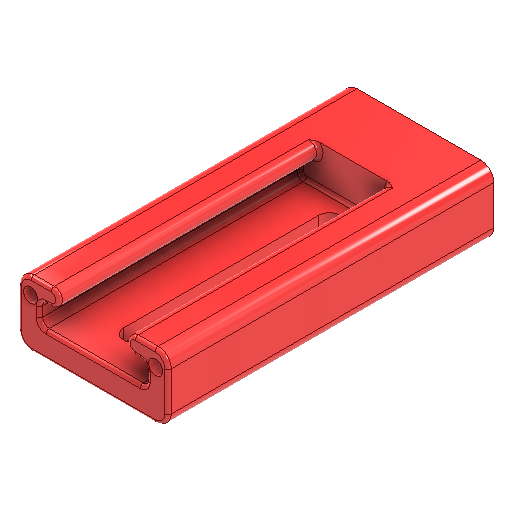
# Autodesk Inventor part: VerticalProfile
Saved by Autodesk Inventor 2023 (Build 270158000, 158)
## iProperties
Created: 2024-05-30
Part Number: VerticalProfile
Material: Generic
Document SubType Name: Modeling
Designer: Sven
Density: 1 g/cm^3
Appearance: Light Red
Author: Sven
Autodesk Inventor part; units mm, degrees
ref_plane "YZ Plane" through (0, 0, 0) normal (1, 0, 0) x (0, 1, 0)
ref_plane "XZ Plane" through (0, 0, 0) normal (0, 1, 0) x (-1, 0, 0)
ref_plane "XY Plane" through (0, 0, 0) normal (0, 0, 1) x (1, 0, 0)
sketch "Sketch1" plane through (0, 0, 0) normal (0, 0, 1) x (1, 0, 0)
  circle A0 centre (-4.5, -25.25) radius 1.65 projected
  circle A1 centre (4.5, -25.25) radius 1.65 projected
  arc A2 (25.5, 29.25) -> (23.5, 31.25) centre (23.5, 29.25) ccw projected
  line L0 (23.5, 31.25) -> (-23.5, 31.25) projected
  arc A3 (-23.5, 31.25) -> (-25.5, 29.25) centre (-23.5, 29.25) ccw projected
  line L1 (-25.5, 29.25) -> (-25.5, -29.25) projected
  arc A4 (-25.5, -29.25) -> (-23.5, -31.25) centre (-23.5, -29.25) ccw projected
  line L2 (-23.5, -31.25) -> (23.5, -31.25) projected
  arc A5 (23.5, -31.25) -> (25.5, -29.25) centre (23.5, -29.25) ccw projected
  line L3 (25.5, -29.25) -> (25.5, 29.25) projected
  line L4 (9.5, -21.25) -> (-9.5, -21.25)
  line L5 (-11.5, -23.25) -> (-11.5, -29.25)
  line L6 (-9.5, -31.25) -> (9.5, -31.25)
  line L7 (11.5, -29.25) -> (11.5, -23.25)
  circle A6 centre (4.5, -25.25) radius 2
  circle A7 centre (-4.5, -25.25) radius 2
  arc A8 (11.5, -23.25) -> (9.5, -21.25) centre (9.5, -23.25) ccw
  arc A9 (-9.5, -21.25) -> (-11.5, -23.25) centre (-9.5, -23.25) ccw
  arc A10 (-11.5, -29.25) -> (-9.5, -31.25) centre (-9.5, -29.25) ccw
  arc A11 (9.5, -31.25) -> (11.5, -29.25) centre (9.5, -29.25) ccw
  circle A12 centre (9.6, -23.75) radius 1.1 projected
  circle A13 centre (-9.6, -23.75) radius 1.1 projected
  point P0 (0, 0)
  point P1 (-11.5, -31.25)
  point P2 (0, -21.25)
  point P3 (0, -31.25)
  dimension "d0" = 23
  dimension "d1" = 10
  dimension "d2" = 4
  dimension "d3" = 4
  dimension "d4" = 2
  dimension "d5" = 2
  constraints: 8 end point, 8 point on circle, 8 tangent, 6 centre point, 3 point on line, 2 coincident, 2 equal radius, 2 midpoint, 2 parallel, 1 horizontal, 1 perpendicular, 1 vertical alignment
  measures "d0" distance between parallel lines of L5 L7
  measures "d1" distance between parallel lines of L6 L4
  measures "d2" diameter of A6
  measures "d3" diameter of A7
  measures "d4" radius of A8
  measures "d5" radius of A9
extrude "Extrusion1" add sketch "Sketch1" along normal blind 6 contours L2 A10 L5 A9 L4 A8 L7 A11 | A12 | A13
sketch "Sketch2" plane through (0, 0, 6) normal (0, 0, 1) x (1, 0, 0)
  arc A0 (-11.5, -29.25) -> (-9.5, -31.25) centre (-9.5, -29.25) ccw projected
  line L0 (-9.5, -31.25) -> (9.5, -31.25) projected
  arc A1 (9.5, -31.25) -> (11.5, -29.25) centre (9.5, -29.25) ccw projected
  line L1 (11.5, -29.25) -> (11.5, -23.25) projected
  arc A2 (11.5, -23.25) -> (9.5, -21.25) centre (9.5, -23.25) ccw projected
  line L2 (9.5, -21.25) -> (-9.5, -21.25) projected
  arc A3 (-9.5, -21.25) -> (-11.5, -23.25) centre (-9.5, -23.25) ccw projected
  line L3 (-11.5, -23.25) -> (-11.5, -29.25) projected
  circle A4 centre (-4.5, -25.25) radius 2 projected
  circle A5 centre (4.5, -25.25) radius 2 projected
  point P0 (0, 0)
extrude "Extrusion2" add sketch "Sketch2" along normal blind 4 contours L3 A3 L2 A2 L1 A1 L0 A0 | A4 | A5
sketch "Sketch3" plane through (0, 0, 10) normal (0, 0, 1) x (1, 0, 0)
  line L0 (9.5, -21.25) -> (-9.5, -21.25) projected
  arc A0 (6.45, -21.25) -> (6.45, -23.75) centre (6.45, -22.5) ccw
  arc A1 (-6.45, -23.75) -> (-6.45, -21.25) centre (-6.45, -22.5) ccw
  line L1 (9.5, -21.25) -> (-9.5, -21.25) projected
  line L2 (6.45, -23.75) -> (-6.45, -23.75)
  line L3 (-9.5, -31.25) -> (9.5, -31.25) projected
  line L4 (7.25, -27.25) -> (-7.25, -27.25)
  line L5 (8.25, -26.25) -> (8.25, -24.75)
  line L6 (11.5, -29.25) -> (11.5, -23.25) projected
  line L7 (-8.25, -26.25) -> (-8.25, -24.75)
  line L8 (-11.5, -23.25) -> (-11.5, -29.25) projected
  line L9 (6.45, -23.75) -> (7.25, -23.75)
  line L10 (-6.45, -23.75) -> (-7.25, -23.75)
  arc A2 (8.25, -24.75) -> (7.25, -23.75) centre (7.25, -24.75) ccw
  arc A3 (7.25, -27.25) -> (8.25, -26.25) centre (7.25, -26.25) ccw
  arc A4 (-8.25, -26.25) -> (-7.25, -27.25) centre (-7.25, -26.25) ccw
  arc A5 (-7.25, -23.75) -> (-8.25, -24.75) centre (-7.25, -24.75) ccw
  line L11 (-9.5, -31.25) -> (9.5, -31.25) projected
  arc A6 (9.5, -31.25) -> (11.5, -29.25) centre (9.5, -29.25) ccw projected
  line L12 (11.5, -29.25) -> (11.5, -23.25) projected
  arc A7 (11.5, -23.25) -> (9.5, -21.25) centre (9.5, -23.25) ccw projected
  line L13 (9.5, -21.25) -> (-9.5, -21.25) projected
  arc A8 (-9.5, -21.25) -> (-11.5, -23.25) centre (-9.5, -23.25) ccw projected
  line L14 (-11.5, -23.25) -> (-11.5, -29.25) projected
  arc A9 (-11.5, -29.25) -> (-9.5, -31.25) centre (-9.5, -29.25) ccw projected
  point P0 (0, 0)
  point P1 (0, -23.75)
  point P2 (0, -31.25)
  point P3 (8.25, -23.75)
  point P4 (-8.25, -23.75)
  dimension "d10" = 1.25
  dimension "d11" = 12.9
  dimension "d12" = 4
  dimension "d13" = 3.25
  dimension "d14" = 3.25
  dimension "d15" = 1
  constraints: 12 end point, 12 point on circle, 8 tangent, 6 centre point, 6 point on line, 5 vertical alignment, 4 equal radius, 2 horizontal, 2 horizontal alignment, 2 midpoint, 2 vertical, 1 collinear, 1 parallel
  measures "d10" radius of A1
  measures "d11" distance of L2.start L2.end
  measures "d12" distance between parallel lines of L3 L4
  measures "d13" distance between parallel lines of L5 L6
  measures "d14" distance between parallel lines of L8 L7
  measures "d15" radius of A2
extrude "Extrusion3" add sketch "Sketch3" along normal blind 40 contours A7 L6 A6 L3 A9 L8 A8 L0 A1 L10 A5 L7 A4 L4 A3 L5 A2 L9 A0
sketch "Sketch4" plane through (0, 0, 50) normal (0, 0, 1) x (1, 0, 0)
  circle A0 centre (9.6, -23.75) radius 1.1
  circle A1 centre (-9.6, -23.75) radius 1.1
  arc A2 (-6.45, -23.75) -> (-6.45, -21.25) centre (-6.45, -22.5) ccw projected
  line L0 (-6.45, -21.25) -> (-9.5, -21.25) projected
  arc A3 (-9.5, -21.25) -> (-11.5, -23.25) centre (-9.5, -23.25) ccw projected
  line L1 (-11.5, -23.25) -> (-11.5, -29.25) projected
  arc A4 (-11.5, -29.25) -> (-9.5, -31.25) centre (-9.5, -29.25) ccw projected
  line L2 (-9.5, -31.25) -> (9.5, -31.25) projected
  arc A5 (9.5, -31.25) -> (11.5, -29.25) centre (9.5, -29.25) ccw projected
  line L3 (11.5, -29.25) -> (11.5, -23.25) projected
  arc A6 (11.5, -23.25) -> (9.5, -21.25) centre (9.5, -23.25) ccw projected
  line L4 (9.5, -21.25) -> (6.45, -21.25) projected
  arc A7 (6.45, -21.25) -> (6.45, -23.75) centre (6.45, -22.5) ccw projected
  line L5 (6.45, -23.75) -> (7.25, -23.75) projected
  arc A8 (8.25, -24.75) -> (7.25, -23.75) centre (7.25, -24.75) ccw projected
  line L6 (8.25, -24.75) -> (8.25, -26.25) projected
  arc A9 (7.25, -27.25) -> (8.25, -26.25) centre (7.25, -26.25) ccw projected
  line L7 (7.25, -27.25) -> (-7.25, -27.25) projected
  arc A10 (-8.25, -26.25) -> (-7.25, -27.25) centre (-7.25, -26.25) ccw projected
  line L8 (-8.25, -26.25) -> (-8.25, -24.75) projected
  arc A11 (-7.25, -23.75) -> (-8.25, -24.75) centre (-7.25, -24.75) ccw projected
  line L9 (-7.25, -23.75) -> (-6.45, -23.75) projected
  line L10 (11.5, -29.25) -> (11.5, -23.25) projected
  line L11 (11.5, -26.25) -> (8.25, -26.25)
  arc A12 (-8.25, -26.25) -> (-7.25, -27.25) centre (-7.25, -26.25) ccw projected
  line L12 (-8.25, -26.25) -> (-11.5, -26.25)
  line L13 (-11.5, -23.25) -> (-11.5, -29.25) projected
  point P0 (0, 0)
  point P1 (9.875, -26.25)
  point P2 (-9.875, -26.25)
  dimension "d18" = 2.2
  dimension "d19" = 2.2
  dimension "d22" = 2.5
  dimension "d34" = 0.275
  dimension "d35" = 0.275
  constraints: 4 end point, 4 midpoint, 2 centre point, 1 horizontal alignment
  measures "d18" diameter of A0
  measures "d19" diameter of A1
  measures "d22" distance from line of L4 A0.centre
  measures "d34" horizontal distance of A0.centre point (9.875, -26.25)
  measures "d35" horizontal distance of A1.centre point (-9.875, -26.25)
extrude "Extrusion4" cut sketch "Sketch4" against normal through all contours A0 | A1
sketch "Sketch5" plane through (-9.5, -31.25, 0) normal (0, -1, 0) x (1, 0, 0)
  line L0 (9.5, 43.75) -> (9.5, 13.75) construction
  line L1 (5.75, 43.75) -> (5.75, 13.75)
  line L2 (13.25, 13.75) -> (13.25, 43.75)
  arc A0 (13.25, 43.75) -> (5.75, 43.75) centre (9.5, 43.75) ccw
  arc A1 (5.75, 13.75) -> (13.25, 13.75) centre (9.5, 13.75) ccw
  line L3 (0, 50) -> (19, 50) projected
  line L4 (0, 0) -> (19, 0) projected
  point P0 (9.5, 0)
  point P1 (9.5, 28.75)
  point P2 (9.5, 50)
  point P3 (9.5, 47.5)
  point P4 (9.5, 0)
  point P5 (9.5, 50)
  dimension "d23" = 7.5
  dimension "d24" = 13.75
  dimension "d25" = 6.25
  constraints: 8 end point, 5 point on circle, 4 midpoint, 4 tangent, 2 centre point, 1 parallel, 1 vertical, 1 vertical alignment
  measures "d23" diameter of A1
  measures "d24" distance of point (9.5, 0) L0.end
  measures "d25" distance of L0.start point (9.5, 50)
extrude "Extrusion5" cut sketch "Sketch5" against normal blind 2
sketch "Sketch6" plane through (-9.5, -29.25, 0) normal (0, -1, 0) x (1, 0, 0)
  arc A0 (5.75, 13.75) -> (13.25, 13.75) centre (9.5, 13.75) ccw projected
  line L0 (13.25, 43.75) -> (13.25, 13.75) projected
  arc A1 (13.25, 43.75) -> (5.75, 43.75) centre (9.5, 43.75) ccw projected
  line L1 (5.75, 13.75) -> (5.75, 43.75) projected
  arc A2 (11.1, 43.75) -> (7.9, 43.75) centre (9.5, 43.75) ccw
  line L2 (11.1, 43.75) -> (11.1, 13.75)
  arc A3 (7.9, 13.75) -> (11.1, 13.75) centre (9.5, 13.75) ccw
  line L3 (7.9, 13.75) -> (7.9, 43.75)
  point P0 (9.5, 0)
  dimension "d28" = 2.15
  constraints: 4 end point, 4 point on circle, 2 centre point, 3 other
  measures "d28" distance between parallel lines of L1 L3
extrude "Extrusion6" cut sketch "Sketch6" against normal through all contours L2 A3 L3 A2
fillet "Fillet1" radius 0.5 8 edges at (0, -31.25, 47.5) (3.75, -31.25, 28.75) (0, -31.25, 10) (-3.75, -31.25, 28.75) (0, -29.25, 47.5) (3.75, -29.25, 28.75) (0, -29.25, 10) (-3.75, -29.25, 28.75)
fillet "Fillet2" radius 0.5 20 edges at (10.9142, -30.6642, 50) (11.5, -26.25, 50) (10.9142, -21.8358, 50) (7.975, -21.25, 50) (5.2, -22.5, 50) (6.85, -23.75, 50) (7.9571, -24.0429, 50) (8.25, -25.5, 50) (7.9571, -26.9571, 50) (0, -27.25, 50) (-7.9571, -26.9571, 50) (-8.25, -25.5, 50) (-7.9571, -24.0429, 50) (-6.85, -23.75, 50) (-5.2, -22.5, 50) (-7.975, -21.25, 50) (-10.9142, -21.8358, 50) (-11.5, -26.25, 50) (-10.9142, -30.6642, 50) (0, -31.25, 50)
fillet "Fillet3" radius 0.5 11 edges at (7.9571, -26.9571, 10) (8.25, -25.5, 10) (7.9571, -24.0429, 10) (6.85, -23.75, 10) (5.2, -22.5, 10) (-7.9571, -26.9571, 10) (-8.25, -25.5, 10) (-7.9571, -24.0429, 10) (-6.85, -23.75, 10) (-5.2, -22.5, 10) (0, -27.25, 10)
equation "\"d14\" = d13"
equation "\"d19\" = d18"
equation "\"d35\" = d34"
body "Solid1"
